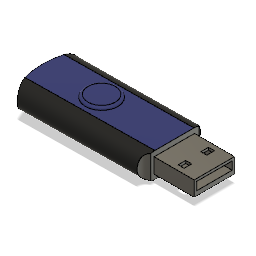
USB v1 (Autodesk Fusion 360 design; units mm, degrees)
Autodesk Fusion 360 part; units mm, degrees
sketch "MASTER SKETCH" plane through (0, 0, 0) normal (0, 1, 0) x (1, 0, 0)
  line L0 (-20.1125, 7.8888) -> (9.6034, 8.2112)
  arc A0 (9.6034, 8.2112) -> (11.0867, 6.3443) centre (11.9278, 8.5352) ccw
  line L1 (11.0867, 6.3443) -> (11.0867, 5.2219)
  line L2 (11.0867, 5.2219) -> (21.1539, 5.2219)
  line L3 (21.1539, 5.2219) -> (21.1539, -4.9577)
  line L4 (21.1539, -4.9577) -> (11.0867, -4.9577)
  line L5 (11.0867, -4.9577) -> (11.0867, -5.8142)
  arc A1 (11.0867, -5.8142) -> (9.8311, -7.945) centre (11.8441, -7.6959) ccw
  line L6 (9.8311, -7.945) -> (-19.9558, -8.3433)
  arc A2 (-20.1125, 7.8888) -> (-19.9558, -8.3433) centre (-3.1266, -0.064) ccw
  line L7 (15.1779, 3.7868) -> (16.7624, 3.7868)
  line L8 (16.7624, 3.7868) -> (16.7624, 1.8338)
  line L9 (16.7624, 1.8338) -> (15.1779, 1.8338)
  line L10 (15.1779, 1.8338) -> (15.1779, 3.7868)
  line L11 (15.1779, -1.2246) -> (16.7624, -1.2246)
  line L12 (16.7624, -1.2246) -> (16.7624, -3.2144)
  line L13 (16.7624, -3.2144) -> (15.1779, -3.2144)
  line L14 (15.1779, -3.2144) -> (15.1779, -1.2246)
  circle A3 centre (-7.2793, 0.4193) radius 4.0763
extrude "Extrude1" add sketch "MASTER SKETCH" along normal blind 6.35 contours L0 A0 L1 L2 L3 L4 L5 A1 L6 A2 | L7 L8 L9 L10 | L11 L12 L13 L14 | A3 in component "BODY"
fillet "Fillet1" radius 3.175 4 edges at (-5.0623, 6.35, 8.1442) (-5.2545, 6.35, -8.05) (-5.0623, 0, 8.1442) (-5.2545, 0, -8.05) in component "BODY"
sketch "Sketch1" plane through (0, 6.35, 0) normal (0, 1, 0) x (-1, 0, 0) in component "BODY"
  line L0 (-21.1539, -5.1613) -> (21.2666, -4.7011)
  arc A0 (21.2666, -4.7011) -> (21.1696, 5.1842) centre (3.1266, 0.064) ccw
  line L1 (21.1696, 5.1842) -> (-21.1539, 4.6184)
  line L2 (-21.1539, 4.6184) -> (-21.1539, -5.1613)
  line L3 (-11.0867, -6.3443) -> (-11.0867, 5.8142)
  line L4 (-11.0867, 5.8142) -> (-21.1539, 5.8142)
  line L5 (-21.1539, 5.8142) -> (-21.1539, -6.3443)
  line L6 (-21.1539, -6.3443) -> (-11.0867, -6.3443)
extrude "Extrude2" cut sketch "Sketch1" against normal blind 1.27 contours L0 L1 L2 L3 L5 | L0 L3 L5 L6 | L1 L3 L4 L5 in component "BODY"
sketch "Sketch2" plane through (0, 0, 0) normal (0, -1, 0) x (1, 0, 0) in component "BODY"
  line L0 (-21.2666, -4.7011) -> (21.1539, -5.1613)
  line L1 (21.1539, -5.1613) -> (21.1539, 4.6184)
  line L2 (21.1539, 4.6184) -> (-21.1696, 5.1842)
  arc A0 (-21.1696, 5.1842) -> (-21.2666, -4.7011) centre (-3.1266, 0.064) ccw
  line L3 (11.0867, 5.8142) -> (11.0867, -6.3443)
  line L4 (11.0867, -6.3443) -> (21.1539, -6.3443)
  line L5 (21.1539, -6.3443) -> (21.1539, 5.8142)
  line L6 (21.1539, 5.8142) -> (11.0867, 5.8142)
extrude "Extrude3" cut sketch "Sketch2" against normal blind 1.27 contours L0 L1 L2 L3 L5 | L0 L3 L4 L5 | L2 L3 L5 L6 in component "BODY"
sketch "Sketch3" plane through (0, 5.08, 0) normal (0, 1, 0) x (-1, 0, 0) in component "BODY"
  line L0 (-21.1539, -5.2219) -> (-11.0867, -5.2219)
  line L1 (-11.0867, -5.2219) -> (-11.0867, 4.9577)
  line L2 (-11.0867, 4.9577) -> (-21.1539, 4.9577)
  line L3 (-21.1539, 4.9577) -> (-21.1539, -5.2219)
  line L4 (-15.8492, -3.9519) -> (-17.3439, -3.9519)
  line L5 (-17.3439, -3.9519) -> (-17.3439, -2.0273)
  line L6 (-17.3439, -2.0273) -> (-15.8492, -2.0273)
  line L7 (-15.8492, -2.0273) -> (-15.8492, -3.9519)
  line L8 (-15.8492, 1.7827) -> (-17.3439, 1.7827)
  line L9 (-17.3439, 1.7827) -> (-17.3439, 3.6681)
  line L10 (-17.3439, 3.6681) -> (-15.8492, 3.6681)
  line L11 (-15.8492, 3.6681) -> (-15.8492, 1.7827)
  dimension "d8" = 3.81
  dimension "d9" = 7.62
  dimension "d10" = 4.7625
  dimension "d11" = 4.7625
  dimension "d12" = 3.81
  dimension "d13" = 3.81
  dimension "d14" = 3.81
  dimension "d15" = 1.27
  dimension "d16" = 6.985
  measures "d8" distance of L6 L8
  measures "d9" distance of L4 L10
  measures "d10" distance of L1 L7
  measures "d11" distance of L1 L11
  measures "d12" distance of L3 L5
  measures "d13" distance of L3 L9
  measures "d14" distance of L6 L8
  measures "d15" distance of L0 L4
  measures "d16" distance of L2 L6
sketch "Sketch4" plane through (21.1539, 0, 0) normal (1, 0, 0) x (0, 0, -1) in component "BODY"
  line L0 (-4.9577, 1.27) -> (5.2219, 1.27)
  line L1 (5.2219, 1.27) -> (5.2219, 5.08)
  line L2 (5.2219, 5.08) -> (-4.9577, 5.08)
  line L3 (-4.9577, 5.08) -> (-4.9577, 1.27)
  line L4 (-4.9577, 5.08) -> (-4.9577, 4.445)
  line L5 (-4.9577, 4.445) -> (-4.3227, 4.445)
  line L6 (5.2219, 5.08) -> (5.2219, 4.445)
  line L7 (5.2219, 4.445) -> (4.5869, 4.445)
  line L8 (4.5869, 4.445) -> (-4.3227, 4.445)
  line L9 (-4.3227, 4.445) -> (-4.3227, 2.413)
  line L10 (-4.3227, 2.413) -> (4.5869, 2.413)
  line L11 (4.5869, 2.413) -> (4.5869, 4.445)
  dimension "d17" = 0.635
  dimension "d18" = 0.635
  dimension "d19" = 0.635
  dimension "d20" = 0.635
  dimension "d21" = 2.032
extrude "Extrude4" cut sketch "Sketch4" against normal blind 11.43 contours L8 L9 L10 L11 in component "BODY"
sketch "Sketch5" plane through (0, 2.413, 0) normal (0, 1, 0) x (-1, 0, 0) in component "BODY"
extrude "Extrude5" cut sketch "Sketch3" against normal blind 1.778 contours L4 L5 L6 L7 | L8 L9 L10 L11 in component "BODY"
sketch "Sketch6" plane through (0, 6.35, 0) normal (0, 1, 0) x (-1, 0, 0) in component "BODY"
  line L0 (-11.0867, 4.753) -> (-11.0867, -5.0521)
  line L1 (-11.0867, -5.0521) -> (21.2666, -4.7011)
  arc A0 (21.2666, -4.7011) -> (21.1696, 5.1842) centre (3.1266, 0.064) ccw
  line L2 (21.1696, 5.1842) -> (-11.0867, 4.753)
  circle A1 centre (7.1973, -0.1496) radius 4.0638
extrude "Extrude6" add sketch "Sketch6" along normal blind 0.635 contours A1 in component "BODY"
sketch "Sketch7" plane through (0, 0, 0) normal (0, -1, 0) x (1, 0, 0) in component "BODY"
  line L0 (11.0867, -5.0521) -> (11.0867, 4.753)
  line L1 (11.0867, 4.753) -> (-21.1696, 5.1842)
  arc A0 (-21.1696, 5.1842) -> (-21.2666, -4.7011) centre (-3.1266, 0.064) ccw
  line L2 (-21.2666, -4.7011) -> (11.0867, -5.0521)
  circle A1 centre (-7.1973, 0) radius 4.0638
extrude "Extrude7" add sketch "Sketch7" along normal blind 0.635 contours A1 in component "BODY"
fillet "Fillet2" radius 0.635 2 edges at (-10.9861, -0.635, -1.4695) (-3.4085, 6.985, -1.6191) 1 faces at (-8.4257, -0.635, 1.6844) in component "BODY"
sketch "Sketch8" plane through (0, 5.08, 0) normal (0, 1, 0) x (-1, 0, 0) in component "BODY"
  line L0 (-17.3439, -3.9519) -> (-17.3439, -2.0273)
  line L1 (-17.3439, -2.0273) -> (-15.8492, -2.0273)
  line L2 (-15.8492, -2.0273) -> (-15.8492, -3.9519)
  line L3 (-15.8492, -3.9519) -> (-17.3439, -3.9519)
  line L4 (-17.3439, 1.7827) -> (-17.3439, 3.6681)
  line L5 (-17.3439, 3.6681) -> (-15.8492, 3.6681)
  line L6 (-15.8492, 3.6681) -> (-15.8492, 1.7827)
  line L7 (-15.8492, 1.7827) -> (-17.3439, 1.7827)
  line L8 (-21.1539, -5.2219) -> (-11.0867, -5.2219)
  line L9 (-11.0867, -5.2219) -> (-11.0867, 4.9577)
  line L10 (-11.0867, 4.9577) -> (-21.1539, 4.9577)
  line L11 (-21.1539, 4.9577) -> (-21.1539, -5.2219)
  line L12 (-15.8492, -3.9519) -> (-17.3439, -3.9519)
  line L13 (-17.3439, -3.9519) -> (-17.3439, -2.0273)
  line L14 (-17.3439, -2.0273) -> (-15.8492, -2.0273)
  line L15 (-15.8492, -2.0273) -> (-15.8492, -3.9519)
  line L16 (-15.8492, 1.7827) -> (-17.3439, 1.7827)
  line L17 (-17.3439, 1.7827) -> (-17.3439, 3.6681)
  line L18 (-17.3439, 3.6681) -> (-15.8492, 3.6681)
  line L19 (-15.8492, 3.6681) -> (-15.8492, 1.7827)
extrude "Extrude8" cut sketch "Sketch8" against normal blind 5.842 contours L0 L1 L2 L3 L12 L13 L14 L15 | L4 L5 L6 L7 L16 L17 L18 L19 in component "BODY"
component "BODY" placed x (1, 0, 0) y (0, 1, 0) z (0, 0, 1) at (0, 0, 0)
